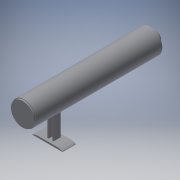
# Autodesk Inventor part: Bevestiging Token Batterij
Saved by Autodesk Inventor 2018.3 (Build 223284000, 284)
## iProperties
Created: 2020-12-14
Part Number: Bevestiging Token Batterij
Material: Generic
Document SubType Name: Modeling
Designer: daanv
Density: 1 g/cm^3
Appearance: Default
Author: daanv
Autodesk Inventor part; units mm, degrees
ref_plane "YZ Plane" through (0, 0, 0) normal (1, 0, 0) x (0, 1, 0)
ref_plane "XZ Plane" through (0, 0, 0) normal (0, 1, 0) x (-1, 0, 0)
ref_plane "XY Plane" through (0, 0, 0) normal (0, 0, 1) x (1, 0, 0)
sketch "Sketch1" plane through (0, 0, 0) normal (0, 0, 1) x (1, 0, 0)
  line L0 (-0.7, 18.5) -> (-2.5, 18.5)
  line L1 (-6.6, 18.5) -> (5.9, 18.5)
  line L2 (5.9, 18.5) -> (5.9, 24)
  line L3 (5.9, 24) -> (-6.6, 24)
  line L4 (-6.6, 24) -> (-6.6, 18.5)
  point P0 (0, 0)
  dimension "d0" = 1.8
  dimension "d2" = 12.5
  dimension "d3" = 5.5
  constraints: 10 end point, 2 parallel, 1 horizontal, 1 perpendicular, 1 point on line
  measures "d0" distance of L0.end L0.start
  measures "d2" distance of L3.end L2.end
  measures "d3" distance of L2.end L1.end
extrude "Extrusion1" add sketch "Sketch1" along normal blind 0.7
sketch "Sketch2" plane through (0, 0, 0.7) normal (0, 0, 1) x (1, 0, 0)
  line L0 (-6.6, 18.5) -> (5.9, 18.5) projected
  line L1 (5.9, 18.5) -> (5.9, 24) projected
  line L2 (5.9, 24) -> (-6.6, 24) projected
  line L3 (-6.6, 24) -> (-6.6, 18.5) projected
  line L4 (-1.6, 22.75) -> (-1.1, 22.75)
  line L5 (-1.1, 22.75) -> (-1.1, 19.75)
  line L6 (-1.1, 19.75) -> (-1.6, 19.75)
  line L7 (-1.6, 19.75) -> (-1.6, 22.75)
  line L8 (0.4, 22.75) -> (0.9, 22.75)
  line L9 (0.9, 22.75) -> (0.9, 19.75)
  line L10 (0.9, 19.75) -> (0.4, 19.75)
  line L11 (0.4, 19.75) -> (0.4, 22.75)
  point P0 (0, 0)
  dimension "d8" = 0.5
  dimension "d9" = 3
  dimension "d10" = 0.5
  dimension "d11" = 1.25
  dimension "d12" = 1.25
  dimension "d13" = 1.5
  dimension "d14" = 5
  dimension "d15" = 5
  constraints: 16 end point, 4 parallel, 2 horizontal, 2 perpendicular, 2 point on line
  measures "d8" distance of L5.end L6.end
  measures "d9" distance of L4.end L5.end
  measures "d10" distance of L9.end L10.end
  measures "d11" distance between parallel lines of L2 L4
  measures "d12" distance between parallel lines of L0 L6
  measures "d13" distance between parallel lines of L11 L5
  measures "d14" distance between parallel lines of L1 L9
  measures "d15" distance between parallel lines of L3 L7
extrude "Extrusion2" add sketch "Sketch2" along normal blind 10 contours L4 L5 L6 L7 | L8 L9 L10 L11
sketch "Sketch4" plane through (-1.6, 19.75, 0.7) normal (0, -1, 0) x (1, 0, 0)
  circle A0 centre (1.25, 14.8) radius 5
  line L0 (-5, 0) -> (7.5, 0) projected
  circle A1 centre (1.25, 14.8) radius 4.9
  point P0 (1.6, -0.7)
  dimension "d35" = 10
  dimension "d36" = 14.8
  dimension "d70" = 9.8
  constraints: 2 centre point, 1 coincident
  measures "d35" diameter of A0
  measures "d36" distance from line of L0 A0.centre
  measures "d70" diameter of A1
extrude "Extrusion4" add sketch "Sketch4" against normal blind 40
sketch "Sketch15" plane through (-0.35, 19.75, 15.5) normal (0, -1, 0) x (1, 0, 0)
  arc A0 (1.25, -4.841229) -> (-1.25, -4.841229) centre (0, 0) ccw
  arc A1 (0.984886, -4.8) -> (-0.984886, -4.8) centre (0, 0) ccw
  line L0 (0.75, -4.8) -> (0.984886, -4.8)
  line L1 (0.75, -4.842262) -> (0.75, -4.8)
  arc A2 (-0.75, -4.842262) -> (0.75, -4.842262) centre (0, 0) ccw
  line L2 (-0.75, -4.842262) -> (-0.75, -4.8)
  line L3 (-0.984886, -4.8) -> (-0.75, -4.8)
  circle A3 centre (0, 0) radius 5
  point P0 (0.35, -15.5)
  constraints: 1 centre point, 1 coincident, 1 concentric
extrude "Extrusion15" add sketch "Sketch15" along normal blind 10
sketch "Sketch16" plane through (-0.35, 9.75, 15.5) normal (0, -1, 0) x (1, 0, 0)
  circle A0 centre (0, 0) radius 5 projected
  point P0 (0.35, -15.5)
extrude "Extrusion16" add sketch "Sketch16" along normal blind 1
chamfer "Chamfer4" distance 4.9 angle 45 1 edges at (-0.35, 9.75, 20.4)
sketch "Sketch17" plane through (-0.35, 59.75, 15.5) normal (0, 1, 0) x (1, 0, 0)
  circle A0 centre (0, 0) radius 5 projected
  point P0 (0.35, 15.5)
extrude "Extrusion17" add sketch "Sketch17" along normal blind 1
chamfer "Chamfer5" distance 4.9 angle 45 1 edges at (-5.25, 59.75, 15.5)
sketch "Sketch18" plane through (-0.35, 60.75, 15.5) normal (0, 1, 0) x (1, 0, 0)
  circle A0 centre (0, 0) radius 5 projected
  circle A1 centre (0, 0) radius 2.4
  point P0 (0.35, 15.5)
  dimension "d83" = 4.8
  constraints: 1 centre point, 1 coincident
  measures "d83" diameter of A1
extrude "Extrusion18" add sketch "Sketch18" along normal blind 3 contours A1
fillet "Fillet4" radius 1.5 1 edges at (-2.75, 60.75, 15.5)
fillet "Fillet5" radius 1.5 1 edges at (-2.75, 63.75, 15.5)
sketch "Sketch19" plane through (-0.35, 8.75, 15.5) normal (0, -1, 0) x (1, 0, 0)
  circle A0 centre (0, 0) radius 5
  circle A1 centre (0, 0) radius 4.774817
  point P0 (0.35, -15.5)
  constraints: 1 centre point, 1 coincident
extrude "Extrusion19" cut sketch "Sketch19" against normal blind 0.1
sketch "Sketch20" plane through (-0.35, 8.75, 15.5) normal (0, -1, 0) x (1, 0, 0)
  circle A0 centre (0, 0) radius 4.774817
  point P0 (0.35, -15.5)
extrude "Extrusion20" add sketch "Sketch20" along normal blind 0.5
chamfer "Chamfer6" distance 0.7 angle 45 2 edges at (5.9, 21.25, 0.7) (-6.6, 21.25, 0.7)
chamfer "Chamfer7" distance 0.7 angle 45 2 edges at (5.2001, 21.25, 0.7) (-5.9001, 21.25, 0.7)
chamfer "Chamfer8" distance 0.7 angle 45 2 edges at (4.5001, 21.25, 0.7) (-5.2001, 21.25, 0.7)
body "Solid1"
